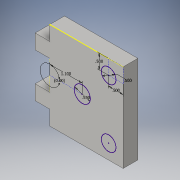
# Autodesk Inventor part: Far End Cap
Saved by Autodesk Inventor 2016 (Build 200138000, 138)
## iProperties
Created: 2016-04-24
Part Number: Far End Cap
Material: Generic
Document SubType Name: Modeling
Designer: rubenjm
Density: 1 g/cm^3
Appearance: Default
Author: rubenjm
Autodesk Inventor part; units mm, degrees
ref_plane "YZ Plane" through (0, 0, 0) normal (1, 0, 0) x (0, 1, 0)
ref_plane "XZ Plane" through (0, 0, 0) normal (0, 1, 0) x (-1, 0, 0)
ref_plane "XY Plane" through (0, 0, 0) normal (0, 0, 1) x (1, 0, 0)
sketch "Sketch1" plane through (0, 0, 0) normal (0, 0, 1) x (1, 0, 0)
  circle A0 centre (27.94, -38.1) radius 6.985 construction
  circle A1 centre (50.8, -12.0577) radius 6.35 construction
  line L0 (63.5, 0.1606) -> (50.8, 0.1606) construction
  line L1 (50.8, 0.1606) -> (50.8, -12.5394) construction
  line L2 (50.8, -12.5394) -> (63.5, -12.5394) construction
  line L3 (63.5, -12.5394) -> (63.5, 0.1606) construction
  circle A2 centre (50.8, -63.5) radius 6.35 construction
  line L4 (16.8275, -31.6842) -> (27.94, -25.2684) construction
  line L5 (27.94, -25.2684) -> (39.0525, -31.6842) construction
  line L6 (39.0525, -31.6842) -> (39.0525, -44.5158) construction
  line L7 (39.0525, -44.5158) -> (27.94, -50.9316) construction
  line L8 (27.94, -50.9316) -> (16.8275, -44.5158) construction
  line L9 (16.8275, -44.5158) -> (16.8275, -31.6842) construction
  line L10 (63.5, 0.1606) -> (0, 0.1606)
  line L11 (0, -76.0394) -> (63.5, -76.0394)
  line L12 (63.5, -76.0394) -> (63.5, 0.1606)
  line L13 (0, -37.9394) -> (-12.7, -37.9394) construction
  line L14 (0, -37.9394) -> (12.7, -37.9394) construction
  line L15 (-12.7, -37.9394) -> (-12.7, 0.1606) construction
  line L16 (-12.7, -12.5394) -> (0, -12.5394)
  line L17 (0, -25.2394) -> (-12.7, -25.2394)
  line L18 (-12.7, -25.2394) -> (-12.7, -12.5394)
  line L19 (0, 0.1606) -> (0, -12.5394)
  line L20 (-12.7, -63.3394) -> (0, -63.3394)
  line L21 (0, -50.6394) -> (-12.7, -50.6394)
  line L22 (-12.7, -50.6394) -> (-12.7, -63.3394)
  line L23 (0, -25.2394) -> (0, -50.6394)
  line L24 (0, -63.3394) -> (0, -76.0394)
  point P0 (0, 0)
  point P1 (0, 0)
  dimension "d0" = 13.97
  dimension "d1" = 12.7
  dimension "d2" = 12.7
  dimension "d3" = 22.225
  dimension "d6" = 63.5
  dimension "d7" = 76.2
  dimension "d13" = 12.7
  dimension "d14" = 180
  dimension "d15" = 38.1
  dimension "d16" = 90
  dimension "d19" = 12.7
  constraints: 50 end point, 10 parallel, 5 horizontal, 4 perpendicular, 4 symmetric about line, 3 centre point, 1 collinear, 1 midpoint
  measures "d0" diameter of A0
  measures "d1" diameter of A1
  measures "d2" distance of L2.end L1.end
  measures "d3" distance between parallel lines of L9 L6
  measures "d6" distance of L11.start L11.end
  measures "d7" distance of L11.start L10.end
  measures "d13" distance of L13.start L13.end
  measures "d14" angle of L13 L14
  measures "d15" distance of L13.end L15.end
  measures "d16" angle of L13 L15
  measures "d19" distance of L17.start L17.end
extrude "Extrusion1" add sketch "Sketch1" along normal blind 12.7
sketch "Sketch3" plane through (0, 0, 12.7) normal (0, 0, 1) x (1, 0, 0)
  line L0 (0, -25.2394) -> (0, -50.6394) construction
  line L1 (0, -37.9394) -> (27.94, -37.9394) construction
  line L2 (0, -37.9394) -> (27.94, -37.9394) construction
  circle A0 centre (27.94, -37.9394) radius 6.985
  line L3 (63.5, 0.1606) -> (0, 0.1606) projected
  line L4 (63.5, 0.1606) -> (50.8, 0.1606) construction
  line L5 (50.8, 0.1606) -> (50.8, -12.5394) construction
  line L6 (50.8, -12.5394) -> (63.5, -12.5394) construction
  line L7 (63.5, -12.5394) -> (63.5, 0.1606) construction
  circle A1 centre (50.8, -12.5394) radius 6.35
  circle A2 centre (50.8, -63.3394) radius 6.35
  point P0 (0, 0)
  dimension "d36" = 27.94
  dimension "d37" = 0
  dimension "d38" = 13.97
  dimension "d41" = 12.7
  dimension "d42" = 12.7
  dimension "d43" = 12.7
  constraints: 12 end point, 3 centre point, 3 horizontal, 2 coincident, 2 parallel, 1 collinear, 1 midpoint, 1 perpendicular, 1 symmetric about line, 1 other
  measures "d36" distance of L1.start L1.end
  measures "d37" distance between parallel lines of L1 L2
  measures "d38" diameter of A0
  measures "d41" distance of L6.end L5.end
  measures "d42" distance of L5.end L4.end
  measures "d43" diameter of A1
body "Solid1"
